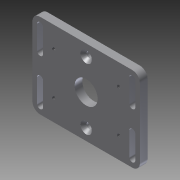
# Autodesk Inventor part: Dewalt Drill Drive CIMmotor Adaptor rectangle
Saved by Autodesk Inventor 2012 (Build 160160000, 160)
## iProperties
Created: 2012-07-04
Part Number: Dewalt Drill Drive CIMmotor Adaptor rectangle
Material: Default
Document SubType Name: Modeling
Designer: Bruce
Density: 1 g/cm^3
Author: Bruce
Autodesk Inventor part; units mm, degrees
ref_plane "YZ Plane" through (0, 0, 0) normal (1, 0, 0) x (0, 1, 0)
ref_plane "XZ Plane" through (0, 0, 0) normal (0, 1, 0) x (-1, 0, 0)
ref_plane "XY Plane" through (0, 0, 0) normal (0, 0, 1) x (1, 0, 0)
sketch "Sketch1" plane through (0, 0, 0) normal (0, 0, 1) x (1, 0, 0)
  circle A0 centre (0, 0) radius 34.925
  circle A1 centre (0, 0) radius 9.525
  line L0 (-44.45, 34.925) -> (44.45, 34.925)
  line L1 (44.45, 34.925) -> (44.45, -34.925)
  line L2 (44.45, -34.925) -> (-44.45, -34.925)
  line L3 (-44.45, -34.925) -> (-44.45, 34.925)
  line L4 (-40.64, 28.575) -> (-35.56, 28.575)
  line L5 (-35.56, 28.575) -> (-35.56, 9.525)
  line L6 (-35.56, 9.525) -> (-40.64, 9.525)
  line L7 (-40.64, 9.525) -> (-40.64, 28.575)
  arc A2 (-35.56, 28.575) -> (-40.64, 28.575) centre (-38.1, 28.575) ccw
  arc A3 (-40.64, 9.525) -> (-35.56, 9.525) centre (-38.1, 9.525) ccw
  line L8 (35.56, 28.575) -> (40.64, 28.575)
  line L9 (40.64, 28.575) -> (40.64, 9.525)
  line L10 (40.64, 9.525) -> (35.56, 9.525)
  line L11 (35.56, 9.525) -> (35.56, 28.575)
  arc A4 (40.64, 28.575) -> (35.56, 28.575) centre (38.1, 28.575) ccw
  arc A5 (35.56, 9.525) -> (40.64, 9.525) centre (38.1, 9.525) ccw
  line L12 (-40.64, -9.525) -> (-35.56, -9.525)
  line L13 (-35.56, -9.525) -> (-35.56, -28.575)
  line L14 (-35.56, -28.575) -> (-40.64, -28.575)
  line L15 (-40.64, -28.575) -> (-40.64, -9.525)
  arc A6 (-35.56, -9.525) -> (-40.64, -9.525) centre (-38.1, -9.525) ccw
  arc A7 (-40.64, -28.575) -> (-35.56, -28.575) centre (-38.1, -28.575) ccw
  line L16 (35.56, -9.525) -> (40.64, -9.525)
  line L17 (40.64, -9.525) -> (40.64, -28.575)
  line L18 (40.64, -28.575) -> (35.56, -28.575)
  line L19 (35.56, -28.575) -> (35.56, -9.525)
  arc A8 (40.64, -9.525) -> (35.56, -9.525) centre (38.1, -9.525) ccw
  arc A9 (35.56, -28.575) -> (40.64, -28.575) centre (38.1, -28.575) ccw
  point P0 (0, 25.4)
  point P1 (0, -25.4)
  point P2 (-26.797, -17.4625)
  point P3 (-26.797, 17.4625)
  point P4 (26.797, 17.4625)
  point P5 (26.797, -17.4625)
  dimension "d0" = 69.85
  dimension "d1" = 19.05
  dimension "d2" = 25.4
  dimension "d3" = 25.4
  dimension "d4" = 26.797
  dimension "d5" = 17.4625
  dimension "d6" = 17.4625
  dimension "d7" = 26.797
  dimension "d24" = 34.925
  dimension "d25" = 69.85
  dimension "d26" = 44.45
  dimension "d28" = 44.45
  dimension "d30" = 5.08
  dimension "d31" = 19.05
  dimension "d33" = 6.35
  dimension "d34" = 6.35
  dimension "d37" = 76.2
  dimension "d40" = 38.1
  constraints: 40 end point, 16 point on circle, 10 centre point, 4 parallel, 4 tangent, 4 vertical alignment, 3 horizontal, 2 coincident, 2 horizontal alignment, 2 perpendicular, 1 vertical, 36 other
  measures "d0" diameter of A0
  measures "d1" diameter of A1
  measures "d2" distance of point (0, 0) point (0, 25.4)
  measures "d3" distance of point (0, -25.4) point (0, 0)
  measures "d4" horizontal distance of point (-26.797, -17.463) point (0, 0)
  measures "d5" vertical distance of point (-26.797, -17.463) point (0, 0)
  measures "d6" vertical distance of point (0, 0) point (-26.797, 17.463)
  measures "d7" horizontal distance of point (26.797, -17.463) point (0, 0)
  measures "d24" distance from line of point (0, 0) L0
  measures "d25" distance of L2.end L0.start
  measures "d26" distance from line of A0.centre L3
  measures "d28" distance from line of L1 point (0, 0)
  measures "d30" distance between parallel lines of L5 L7
  measures "d31" distance of L6.end L4.start
  measures "d33" distance from line of L3 A2.centre
  measures "d34" distance between parallel lines of L0 L4
  measures "d37" distance of L5.end L10.start
  measures "d40" distance of L5.end L14.start
extrude "Extrusion1" add sketch "Sketch1" against normal blind 6.35 contours A0
hole "Hole1" at (-26.797, -17.4625, 0) at (-26.797, 17.4625, 0) at (26.797, 17.4625, 0) at (26.797, -17.4625, 0) direction (0, 0, -1) diameter 2.6416 end through all thread size "6-32 UNC" class "2B" standard "ANSI Unified Screw Threads"
hole "Hole2" at (0, 25.4, 0) at (0, -25.4, 0) direction (0, 0, -1) diameter 4.826 end through all countersink diameter 9.525 countersink angle 82
extrude "Extrusion2" add sketch "Sketch1" against normal blind 6.35 contours A0 L0 L1 L2 | A0 L2 L3 L0
fillet "Fillet1" radius 6.35 4 edges at (-44.45, 34.925, -3.175) (44.45, 34.925, -3.175) (44.45, -34.925, -3.175) (-44.45, -34.925, -3.175)
equation "\"d28\" = d26"
body "Solid1"
